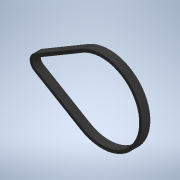
# Autodesk Inventor part: Belt
Saved by Autodesk Inventor 2020 (Build 240168000, 168)
## iProperties
Created: 2019-06-24
Part Number: Belt
Material: Rubber
Document SubType Name: Modeling
Designer: Connor
Density: 0.93 g/cm^3
Appearance: Rubber - Black
Author: Connor
Autodesk Inventor part; units mm, degrees
ref_plane "YZ Plane" through (0, 0, 0) normal (1, 0, 0) x (0, 1, 0)
ref_plane "XZ Plane" through (0, 0, 0) normal (0, 1, 0) x (-1, 0, 0)
ref_plane "XY Plane" through (0, 0, 0) normal (0, 0, 1) x (1, 0, 0)
sketch "Sketch1" plane through (0, 0, 0) normal (0, 0, 1) x (1, 0, 0)
  circle A0 centre (0, 0) radius 9.55 construction
  circle A1 centre (75.05, 0) radius 47.745 construction
  line L0 (-4.8603, 8.2207) -> (50.7513, 41.0993)
  line L1 (-4.8603, -8.2207) -> (50.7513, -41.0993)
  arc A2 (-4.8603, 8.2207) -> (-4.8603, -8.2207) centre (0, 0) ccw
  arc A3 (50.7513, -41.0993) -> (50.7513, 41.0993) centre (75.05, 0) ccw
  line L2 (52.2501, 38.5643) -> (-3.3615, 5.6856)
  arc A4 (-3.3615, 5.6856) -> (-3.3615, -5.6856) centre (0, 0) ccw
  line L3 (-3.3615, -5.6856) -> (52.2501, -38.5643)
  arc A5 (52.2501, -38.5643) -> (52.2501, 38.5643) centre (75.05, 0) ccw
  line L4 (50.311, 41.8439) -> (-5.3005, 8.9653)
  arc A6 (-5.3005, 8.9653) -> (-5.3005, -8.9653) centre (0, 0) ccw
  line L5 (-5.3005, -8.9653) -> (50.311, -41.8439)
  arc A7 (50.311, -41.8439) -> (50.311, 41.8439) centre (75.05, 0) ccw
  dimension "d0" = 19.1
  dimension "d1" = 95.49
  dimension "d2" = 75.05
  dimension "d6" = 2.945
  dimension "d7" = 3.81
  constraints: 16 point on circle, 12 end point, 8 centre point, 4 tangent, 3 coincident, 1 horizontal alignment, 6 other
  measures "d0" diameter of A0
  measures "d1" diameter of A1
  measures "d2" distance of A1.centre point (0, 0)
  measures "d6" distance between parallel lines of L2 L0
  measures "d7" distance between parallel lines of L2 L4
extrude "Extrusion1" add sketch "Sketch1" along normal blind 9 contours L0 A3 L1 A2 | A7 L5 A6 L4
body "Solid1"
